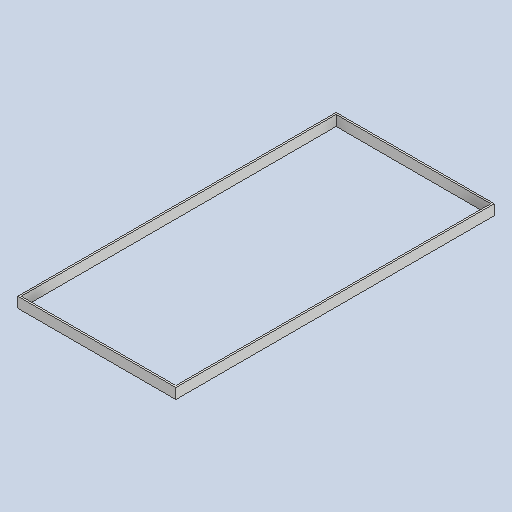
# Autodesk Inventor part: Back rubber bands
Saved by Autodesk Inventor 2022 (Build 260153070, 153G)
## iProperties
Created: 2021-09-05
Part Number: Back rubber bands
Material: Generic
Document SubType Name: Modeling
Designer: Main Account
Density: 1 g/cm^3
Appearance: Default
Author: Main Account
Autodesk Inventor part; units mm, degrees
ref_plane "YZ Plane" through (0, 0, 0) normal (1, 0, 0) x (0, 1, 0)
ref_plane "XZ Plane" through (0, 0, 0) normal (0, 1, 0) x (-1, 0, 0)
ref_plane "XY Plane" through (0, 0, 0) normal (0, 0, 1) x (1, 0, 0)
sketch "Sketch1" plane through (0, 0, 0) normal (1, 0, 0) x (0, 1, 0)
  line L0 (0, 0) -> (4.7625, 0)
  line L1 (4.7625, 0) -> (4.7625, -145.796)
  line L2 (4.7625, -145.796) -> (0, -145.796)
  line L3 (0, -145.796) -> (0, 0)
  dimension "d1" = 4.7625
  dimension "d2" = 145.796
  constraints: 8 end point, 2 parallel, 1 horizontal, 1 perpendicular
  measures "d1" distance of L1.end L2.end
  measures "d2" distance of L0.end L1.end
extrude "Extrusion1" add sketch "Sketch1" along normal blind 0.7937
sketch "Sketch2" plane through (0, 0, -145.796) normal (0, 0, -1) x (-1, 0, 0)
  line L0 (-0.7937, 0) -> (-0.7937, 4.7625) projected
  line L1 (-0.7937, 0) -> (71.5963, 0)
  line L2 (71.5963, 0) -> (71.5963, 4.7625)
  line L3 (71.5963, 4.7625) -> (-0.7937, 4.7625)
  line L4 (-0.7937, 4.7625) -> (-0.7937, 0)
  point P0 (0, 0)
  dimension "d5" = 72.39
  dimension "d6" = 4.7625
  constraints: 8 end point, 2 parallel, 1 horizontal, 1 perpendicular
  measures "d5" distance of L3.end L2.end
  measures "d6" distance of L2.end L1.end
extrude "Extrusion2" add sketch "Sketch2" against normal blind 0.7937
sketch "Sketch3" plane through (-71.5963, 0, -145.796) normal (-1, 0, 0) x (0, 0, 1)
  line L0 (145.796, 4.7625) -> (145.796, 0) projected
  line L1 (0, 0) -> (145.796, 0)
  line L2 (145.796, 0) -> (145.796, 4.7625)
  line L3 (145.796, 4.7625) -> (0, 4.7625)
  line L4 (0, 4.7625) -> (0, 0)
  constraints: 8 end point, 2 parallel, 1 horizontal, 1 perpendicular
extrude "Extrusion3" add sketch "Sketch3" against normal blind 0.7937
sketch "Sketch4" plane through (-71.5963, 0, 0) normal (0, 0, 1) x (1, 0, 0)
  line L0 (0, 0) -> (0, 4.7625) projected
  line L1 (71.5963, 4.7625) -> (72.39, 4.7625) projected
  line L2 (0, 0) -> (72.39, 0)
  line L3 (72.39, 0) -> (72.39, 4.7625)
  line L4 (72.39, 4.7625) -> (0, 4.7625)
  line L5 (0, 4.7625) -> (0, 0)
  point P0 (71.5963, 0)
  constraints: 8 end point, 2 parallel, 1 horizontal, 1 perpendicular
extrude "Extrusion4" add sketch "Sketch4" against normal blind 0.7937
body "Solid1"
